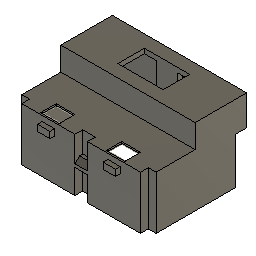
blankCoverWithRecess2Wide (Autodesk Fusion 360 design; units mm, degrees)
part number: 2026-01-13-17-30-06-781
Autodesk Fusion 360 part; units mm, degrees
sketch "Skizze1" plane through (0, 0, 0) normal (0, 0, 1) x (1, 0, 0)
  line L0 (21.5, 12.75) -> (21.5, -12.75)
  line L1 (-21.5, -12.75) -> (-21.5, 12.75)
  line L2 (1.75, 0) -> (22.5, 0)
  line L3 (0, 1.75) -> (0, 22.5)
  line L4 (-21.5, 12.75) -> (-19, 12.75)
  line L5 (-19, 12.75) -> (-19, 15.25)
  line L6 (19, 15.25) -> (19, 12.75)
  line L7 (19, 12.75) -> (21.5, 12.75)
  line L8 (-21.5, -12.75) -> (-19, -12.75)
  line L9 (-19, -12.75) -> (-19, -15.25)
  line L10 (19, -15.25) -> (19, -12.75)
  line L11 (19, -12.75) -> (21.5, -12.75)
  line L12 (2, -15.25) -> (2, -12.75)
  line L13 (2, -12.75) -> (-2, -12.75)
  line L14 (-2, -12.75) -> (-2, -15.25)
  line L15 (2, 15.25) -> (2, 12.75)
  line L16 (2, 12.75) -> (-2, 12.75)
  line L17 (-2, 12.75) -> (-2, 15.25)
  line L18 (-19, 15.25) -> (-2, 15.25)
  line L19 (2, 15.25) -> (19, 15.25)
  line L20 (19, -15.25) -> (2, -15.25)
  line L21 (-2, -15.25) -> (-19, -15.25)
  dimension "d1" = 43
  dimension "d4" = 2.5
  dimension "d5" = 2.5
  dimension "d6" = 2.5
  dimension "d7" = 2.5
  dimension "d8" = 30.5
  dimension "d9" = 2.5
  dimension "d10" = 2.5
  dimension "d11" = 2.5
  dimension "d12" = 2.5
  dimension "d13" = 17
  dimension "d14" = 17
  dimension "d15" = 2.5
  constraint vertical L0
  constraint vertical L1
  constraint symmetric L0 L1 L3
  constraint coincident L1 L4.start
  constraint perpendicular L1 L4
  constraint perpendicular L4 L5
  constraint coincident L0 L7.end
  constraint perpendicular L0 L7
  constraint coincident L1.end L4.start
  constraint perpendicular L1 L8
  constraint perpendicular L8 L9
  constraint coincident L0 L11.end
  constraint perpendicular L0 L11
  constraint coincident L0.end L11.end
  constraint coincident L0.start L7.end
  constraint vertical L12
  constraint horizontal L13
  constraint vertical L14
  constraint vertical L15
  constraint horizontal L16
  constraint vertical L17
  constraint perpendicular L17 L18
  constraint perpendicular L6 L19
  constraint perpendicular L12 L20
  constraint perpendicular L9 L21
  constraint vertical L6
  constraint perpendicular L10 L20
  constraint symmetric L2 L19 L20
  constraint symmetric L2 L18 L21
  constraint equal L18 L21
  constraint equal L19 L20
  constraint equal L12 L15
  constraint equal L0 L1
  measures "d1" distance of L1.end L0.start
  measures "d4" distance of L4.end L5.end
  measures "d5" distance of L1.end L4.end
  measures "d6" distance of L8.end L9.end
  measures "d7" distance of L1.start L8.end
  measures "d8" distance of L5.end L9.end
  measures "d9" distance of L10.end L0.end
  measures "d10" distance of L10.start L10.end
  measures "d11" distance of L6.end L0.start
  measures "d12" distance of L6.start L6.end
  measures "d13" distance of L9.end L14.end
  measures "d14" distance of L10.start L12.start
  measures "d15" distance of L12.start L12.end
extrude "Extrusion1" add sketch "Skizze1" along normal blind 23 thin wall 1.5 inside
sketch "Skizze3" plane through (0, 0, 23) normal (0, 0, 1) x (-1, 0, 0)
  line L0 (-17.5, 13.75) -> (-3.5, 13.75)
  line L1 (-3.5, 13.75) -> (-3.5, 11.25)
  line L2 (-3.5, 11.25) -> (3.5, 11.25)
  line L3 (3.5, 11.25) -> (3.5, 13.75)
  line L4 (3.5, 13.75) -> (17.5, 13.75)
  line L5 (17.5, 13.75) -> (17.5, 11.25)
  line L6 (17.5, 11.25) -> (20, 11.25)
  line L7 (20, 11.25) -> (20, -11.25)
  line L8 (20, -11.25) -> (17.5, -11.25)
  line L9 (17.5, -11.25) -> (17.5, -13.75)
  line L10 (17.5, -13.75) -> (3.5, -13.75)
  line L11 (3.5, -13.75) -> (3.5, -11.25)
  line L12 (3.5, -11.25) -> (-3.5, -11.25)
  line L13 (-3.5, -11.25) -> (-3.5, -13.75)
  line L14 (-3.5, -13.75) -> (-17.5, -13.75)
  line L15 (-17.5, -13.75) -> (-17.5, -11.25)
  line L16 (-17.5, -11.25) -> (-20, -11.25)
  line L17 (-20, -11.25) -> (-20, 11.25)
  line L18 (-20, 11.25) -> (-17.5, 11.25)
  line L19 (-17.5, 11.25) -> (-17.5, 13.75)
  line L20 (-19, 15.25) -> (-19, 12.75)
  line L21 (-19, 12.75) -> (-21.5, 12.75)
  line L22 (-21.5, 12.75) -> (-21.5, -12.75)
  line L23 (-21.5, -12.75) -> (-19, -12.75)
  line L24 (-19, -12.75) -> (-19, -15.25)
  line L25 (-19, -15.25) -> (-2, -15.25)
  line L26 (-2, -15.25) -> (-2, -12.75)
  line L27 (-2, -12.75) -> (2, -12.75)
  line L28 (2, -12.75) -> (2, -15.25)
  line L29 (2, -15.25) -> (19, -15.25)
  line L30 (19, -15.25) -> (19, -12.75)
  line L31 (19, -12.75) -> (21.5, -12.75)
  line L32 (21.5, -12.75) -> (21.5, 12.75)
  line L33 (21.5, 12.75) -> (19, 12.75)
  line L34 (19, 12.75) -> (19, 15.25)
  line L35 (19, 15.25) -> (2, 15.25)
  line L36 (2, 15.25) -> (2, 12.75)
  line L37 (2, 12.75) -> (-2, 12.75)
  line L38 (-2, 12.75) -> (-2, 15.25)
  line L39 (-2, 15.25) -> (-19, 15.25)
  line L40 (21.5, -16.25) -> (-21.5, -16.25)
  line L41 (-21.5, -16.25) -> (-21.5, 0.25)
  line L42 (-21.5, 0.25) -> (21.5, 0.25)
  line L43 (21.5, 0.25) -> (21.5, -16.25)
  dimension "d20" = 1
  dimension "d21" = 16.5
  constraint horizontal L40
  constraint vertical L41
  constraint horizontal L42
  constraint vertical L43
  constraint coincident L22 L41.end
  constraint coincident L32 L42.end
  measures "d20" distance of L29 L40
  measures "d21" distance of L40 L42
extrude "Extrusion2" add sketch "Skizze3" along normal blind 1.5 contours L7 L8 L9 L10 L11 L12 L13 L14 L15 L16 L17 L42 | L7 L8 L9 L10 L11 L12 L13 L14 L15 L16 L17 L22 L23 L24 L25 L26 L27 L28 L29 L30 L31 L32 L41 L42 L43 | L23 L24 L25 L26 L27 L28 L29 L30 L31 L40 L41 L43
sketch "Skizze4" plane through (21.5, 0, 0) normal (1, 0, 0) x (0, 1, 0)
  line L0 (-12.75, 0) -> (12.75, 0)
  line L1 (12.75, 0) -> (12.75, 23)
  line L2 (12.75, 23) -> (16.25, 23)
  line L3 (16.25, 23) -> (16.25, 24.5)
  line L4 (16.25, 24.5) -> (-0.25, 24.5)
  line L5 (-0.25, 24.5) -> (-0.25, 23)
  line L6 (-0.25, 23) -> (-12.75, 23)
  line L7 (-12.75, 23) -> (-12.75, 0)
  line L8 (-0.25, 23) -> (-15.25, 23)
  line L9 (-15.25, 23) -> (-15.25, 17)
  line L10 (-15.25, 17) -> (-0.25, 17)
  line L11 (-0.25, 17) -> (-0.25, 23)
  line L12 (-15.25, 0) -> (-15.25, 23)
  dimension "d24" = 6
  constraint horizontal L8
  constraint vertical L9
  constraint horizontal L10
  constraint vertical L11
  constraint coincident L9.end L12
  constraint coincident L5.end L6.start
  measures "d24" distance of L5.end L10.end
extrude "Extrusion3" cut sketch "Skizze4" against normal blind 45 contours L7 L8 L9 L10 L12 | L6 L7 L8 L10 L11
sketch "Skizze5" plane through (0, 0, 17) normal (0, 0, 1) x (-1, 0, 0)
  line L0 (2, 15.25) -> (2, 12.75)
  line L1 (2, 12.75) -> (-2, 12.75)
  line L2 (-2, 12.75) -> (-2, 15.25)
  line L3 (-2, 15.25) -> (-19, 15.25)
  line L4 (-19, 15.25) -> (-19, 12.75)
  line L5 (-19, 12.75) -> (-21.5, 12.75)
  line L6 (-21.5, 12.75) -> (-21.5, 0.25)
  line L7 (-21.5, 0.25) -> (-20, 0.25)
  line L8 (-20, 0.25) -> (-20, 11.25)
  line L9 (-20, 11.25) -> (-17.5, 11.25)
  line L10 (-17.5, 11.25) -> (-17.5, 13.75)
  line L11 (-17.5, 13.75) -> (-3.5, 13.75)
  line L12 (-3.5, 13.75) -> (-3.5, 11.25)
  line L13 (-3.5, 11.25) -> (3.5, 11.25)
  line L14 (3.5, 11.25) -> (3.5, 13.75)
  line L15 (3.5, 13.75) -> (17.5, 13.75)
  line L16 (17.5, 13.75) -> (17.5, 11.25)
  line L17 (17.5, 11.25) -> (20, 11.25)
  line L18 (20, 11.25) -> (20, 0.25)
  line L19 (20, 0.25) -> (21.5, 0.25)
  line L20 (21.5, 0.25) -> (21.5, 12.75)
  line L21 (21.5, 12.75) -> (19, 12.75)
  line L22 (19, 12.75) -> (19, 15.25)
  line L23 (19, 15.25) -> (2, 15.25)
  line L24 (20, 0.25) -> (20, 11.25)
  line L25 (17.5, 11.25) -> (17.5, 13.75)
  line L26 (3.5, 13.75) -> (17.5, 13.75)
  line L27 (3.5, 11.25) -> (3.5, 13.75)
  line L28 (3.5, 11.25) -> (-3.5, 11.25)
  line L29 (-3.5, 11.25) -> (-3.5, 13.75)
  line L30 (-3.5, 13.75) -> (-17.5, 13.75)
  line L31 (-17.5, 11.25) -> (-17.5, 13.75)
  line L32 (-17.5, 11.25) -> (-20, 11.25)
  line L33 (-20, 11.25) -> (-20, 0.25)
  line L34 (-20, 0.25) -> (20, 0.25)
  constraint coincident L18.end L19.start
  constraint coincident L17.end L18.start
  constraint coincident L16.end L17.start
  constraint coincident L15.end L16.start
  constraint coincident L14.end L15.start
  constraint coincident L13.end L14.start
  constraint coincident L12.end L13.start
  constraint coincident L11.end L12.start
  constraint coincident L10.end L11.start
  constraint coincident L9.end L10.start
  constraint coincident L8.end L9.start
  constraint coincident L7.end L8.start
extrude "Extrusion4" add sketch "Skizze5" against normal blind 1.5 contours L8 L9 L10 L11 L12 L13 L14 L15 L16 L17 L18 L24 L25 L26 L27 L28 L29 L30 L31 L32 L33 L34
sketch "Skizze6" plane through (0, 0, 23) normal (0, 0, -1) x (1, 0, 0)
  line L0 (-20, 0.25) -> (-20, -11.25)
  line L1 (-20, -11.25) -> (-17.5, -11.25)
  line L2 (-17.5, -11.25) -> (-17.5, -13.75)
  line L3 (-17.5, -13.75) -> (-3.5, -13.75)
  line L4 (-3.5, -13.75) -> (-3.5, -11.25)
  line L5 (-3.5, -11.25) -> (3.5, -11.25)
  line L6 (3.5, -11.25) -> (3.5, -13.75)
  line L7 (3.5, -13.75) -> (17.5, -13.75)
  line L8 (17.5, -13.75) -> (17.5, -11.25)
  line L9 (17.5, -11.25) -> (20, -11.25)
  line L10 (20, -11.25) -> (20, 0.25)
  line L11 (20, 0.25) -> (-20, 0.25)
  line L12 (-20, 0.25) -> (20, 0.25)
  line L13 (20, 0.25) -> (20, -1.25)
  line L14 (20, -1.25) -> (-20, -1.25)
  line L15 (-20, -1.25) -> (-20, 0.25)
  dimension "d29" = 1.5
  constraint horizontal L12
  constraint vertical L13
  constraint horizontal L14
  constraint vertical L15
  constraint coincident L10 L13.end
  constraint coincident L0.start L11.end
  measures "d29" distance of L10.end L13.end
extrude "Extrusion5" add sketch "Skizze6" along normal blind 7.5 contours L0 L10 L11 L12 L13 L14 L15
sketch "Skizze7" plane through (0, 12.75, 0) normal (0, 1, 0) x (-1, 0, 0)
  line L0 (-2, 0) -> (2, 0)
  line L1 (2, 0) -> (2, 23)
  line L2 (2, 23) -> (-2, 23)
  line L3 (-2, 23) -> (-2, 0)
  line L4 (-2, 7.8) -> (2, 7.8)
  line L5 (2, 7.8) -> (2, 10.3)
  line L6 (2, 10.3) -> (-2, 10.3)
  line L7 (-2, 10.3) -> (-2, 7.8)
  dimension "d32" = 7.8
  dimension "d33" = 2.5
  constraint horizontal L4
  constraint vertical L5
  constraint horizontal L6
  constraint vertical L7
  constraint coincident L1 L5.end
  constraint coincident L3 L4.start
  measures "d32" distance of L0 L4
  measures "d33" distance of L4.end L5.end
extrude "Extrusion6" add sketch "Skizze7" along normal blind 2.5 contours L1 L3 L4 L5 L6 L7
chamfer "Fase1" distance 1.5 angle 45 1 edges at (0, 15.25, 10.3)
sketch "Skizze8" plane through (0, -12.75, 0) normal (0, -1, 0) x (1, 0, 0)
  line L0 (2, 17) -> (-2, 17)
  line L1 (-2, 17) -> (-2, 0)
  line L2 (-2, 0) -> (2, 0)
  line L3 (2, 0) -> (2, 17)
  line L4 (-2, 7.8) -> (2, 7.8)
  line L5 (2, 7.8) -> (2, 10.3)
  line L6 (2, 10.3) -> (-2, 10.3)
  line L7 (-2, 10.3) -> (-2, 7.8)
  dimension "d37" = 7.8
  dimension "d38" = 2.5
  constraint horizontal L4
  constraint vertical L5
  constraint horizontal L6
  constraint vertical L7
  constraint coincident L3 L5.end
  constraint coincident L1 L4.start
  measures "d37" distance of L2 L4
  measures "d38" distance of L4.end L5.end
extrude "Extrusion7" add sketch "Skizze8" along normal blind 2.5 contours L1 L3 L4 L5 L6 L7
chamfer "Fase2" distance 1.5 angle 45 1 edges at (0, -15.25, 10.3)
sketch "Skizze9" plane through (0, 0, 23) normal (0, 0, -1) x (1, 0, 0)
  line L0 (20, -1.25) -> (-20, -1.25)
  line L1 (-20, -1.25) -> (-20, -11.25)
  line L2 (-20, -11.25) -> (-17.5, -11.25)
  line L3 (-17.5, -11.25) -> (-17.5, -13.75)
  line L4 (-17.5, -13.75) -> (-3.5, -13.75)
  line L5 (-3.5, -13.75) -> (-3.5, -11.25)
  line L6 (-3.5, -11.25) -> (3.5, -11.25)
  line L7 (3.5, -11.25) -> (3.5, -13.75)
  line L8 (3.5, -13.75) -> (17.5, -13.75)
  line L9 (17.5, -13.75) -> (17.5, -11.25)
  line L10 (17.5, -11.25) -> (20, -11.25)
  line L11 (20, -11.25) -> (20, -1.25)
  line L12 (-7.25, -12.25) -> (7.25, -12.25)
  line L13 (7.25, -12.25) -> (7.25, -3.75)
  line L14 (7.25, -3.75) -> (-7.25, -3.75)
  line L15 (-7.25, -3.75) -> (-7.25, -12.25)
  line L16 (-21.5, -16.25) -> (21.5, -16.25)
  dimension "d42" = 14.5
  dimension "d43" = 12.75
  dimension "d46" = 8.5
  dimension "d47" = 4
  constraint horizontal L12
  constraint vertical L13
  constraint horizontal L14
  constraint vertical L15
  constraint coincident L13.end L14.start
  measures "d42" distance of L13.end L14.end
  measures "d43" distance of L1 L15
  measures "d46" distance of L12.end L13.end
  measures "d47" distance of L12 L16
extrude "Extrusion8" cut sketch "Skizze9" against normal blind 2 contours L5 L6 L7 L12 | L5 L6 L7 L12 L13 L14 L15
extrude "Extrusion9" cut sketch "Skizze9" along normal blind 8 contours L5 L6 L7 L12
chamfer "Fase3" distance 4 distance2 1 1 edges at (0, 11.25, 15) measured on face at (-1.1667, 11.25, 10)
extrude "Extrusion10" add 1 faces at (-20.6667, 14.75, 23) along direction (0, 0, -1) blind 8.2
sketch "Skizze10" plane through (0, -15.25, 0) normal (0, -1, 0) x (1, 0, 0)
  line L0 (-2, 8.8) -> (-2, 17)
  line L1 (-2, 17) -> (-19, 17)
  line L2 (-19, 17) -> (-19, 0)
  line L3 (-19, 0) -> (-2, 0)
  line L4 (-2, 0) -> (-2, 7.8)
  line L5 (-2, 7.8) -> (2, 7.8)
  line L6 (2, 7.8) -> (2, 0)
  line L7 (2, 0) -> (19, 0)
  line L8 (19, 0) -> (19, 17)
  line L9 (19, 17) -> (2, 17)
  line L10 (2, 17) -> (2, 8.8)
  line L11 (2, 8.8) -> (-2, 8.8)
  line L12 (-12.5, 15.3) -> (-8.5, 15.3)
  line L13 (-8.5, 15.3) -> (-8.5, 13.3)
  line L14 (-8.5, 13.3) -> (-12.5, 13.3)
  line L15 (-12.5, 13.3) -> (-12.5, 15.3)
  line L16 (8.5, 15.3) -> (12.5, 15.3)
  line L17 (12.5, 15.3) -> (12.5, 13.3)
  line L18 (12.5, 13.3) -> (8.5, 13.3)
  line L19 (8.5, 13.3) -> (8.5, 15.3)
  dimension "d54" = 4
  dimension "d55" = 2
  dimension "d56" = 2
  dimension "d57" = 4
  dimension "d58" = 6.5
  dimension "d59" = 13.3
  dimension "d60" = 13.3
  dimension "d61" = 6.5
  constraint horizontal L12
  constraint vertical L13
  constraint horizontal L14
  constraint vertical L15
  constraint horizontal L16
  constraint vertical L17
  constraint horizontal L18
  constraint vertical L19
  measures "d54" distance of L12.start L12.end
  measures "d55" distance of L12.end L13.end
  measures "d56" distance of L16.start L18.end
  measures "d57" distance of L16.start L16.end
  measures "d58" distance of L10 L19
  measures "d59" distance of L7 L18
  measures "d60" distance of L3 L14
  measures "d61" distance of L0 L13
extrude "Extrusion11" add sketch "Skizze10" along normal blind 1.5 contours L12 L13 L14 L15 | L16 L17 L18 L19
sketch "Skizze12" plane through (0, 0, 15.5) normal (0, 0, -1) x (1, 0, 0)
  line L0 (20, 11.25) -> (17.5, 11.25)
  line L1 (17.5, 11.25) -> (17.5, 13.75)
  line L2 (17.5, 13.75) -> (3.5, 13.75)
  line L3 (3.5, 13.75) -> (3.5, 11.25)
  line L4 (3.5, 11.25) -> (-3.5, 11.25)
  line L5 (-3.5, 11.25) -> (-3.5, 13.75)
  line L6 (-3.5, 13.75) -> (-17.5, 13.75)
  line L7 (-17.5, 13.75) -> (-17.5, 11.25)
  line L8 (-17.5, 11.25) -> (-20, 11.25)
  line L9 (-20, 11.25) -> (-20, -1.25)
  line L10 (-20, -1.25) -> (20, -1.25)
  line L11 (20, -1.25) -> (20, 11.25)
  line L12 (13.5, 13.75) -> (7.5, 13.75)
  line L13 (7.5, 13.75) -> (7.5, 9.75)
  line L14 (7.5, 9.75) -> (13.5, 9.75)
  line L15 (13.5, 9.75) -> (13.5, 13.75)
  line L16 (-7.5, 13.75) -> (-13.5, 13.75)
  line L17 (-13.5, 13.75) -> (-13.5, 9.75)
  line L18 (-13.5, 9.75) -> (-7.5, 9.75)
  line L19 (-7.5, 9.75) -> (-7.5, 13.75)
  dimension "d70" = 6
  dimension "d71" = 4
  dimension "d72" = 4
  dimension "d73" = 6
  dimension "d74" = 4
  dimension "d75" = 4
  constraint horizontal L12
  constraint vertical L13
  constraint horizontal L14
  constraint vertical L15
  constraint coincident L2 L12.start
  constraint horizontal L16
  constraint vertical L17
  constraint horizontal L18
  constraint vertical L19
  constraint coincident L6 L16.start
  measures "d70" distance of L13.end L14.end
  measures "d71" distance of L12.start L14.end
  measures "d72" distance of L16.start L18.end
  measures "d73" distance of L17.end L18.end
  measures "d74" horizontal distance of L0.end L14.end
  measures "d75" horizontal distance of L7.end L17.end
extrude "Extrusion13" cut sketch "Skizze12" against normal blind 2 contours L2 L12 L13 L14 L15 | L6 L16 L17 L18 L19
fillet "Abrundung1" radius 1 8 edges at (-7.5, -11.75, 15.5) (-10.5, -9.75, 15.5) (-13.5, -11.75, 15.5) (10.5, -9.75, 15.5) (7.5, -11.75, 15.5) (13.5, -11.75, 15.5) (10.5, -13.75, 17) (-10.5, -13.75, 17)
